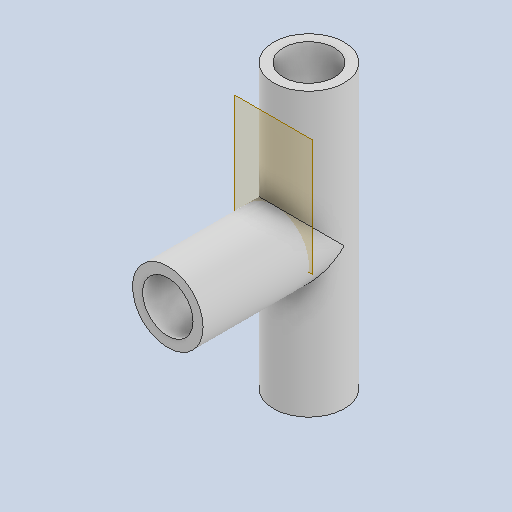
# Autodesk Inventor part: T-joint
Saved by Autodesk Inventor 2025 (Build 290162000, 162)
## iProperties
Created: 2025-07-16
Part Number: T-joint
Material: Generic
Document SubType Name: Modeling
Designer: Pravoslav
Density: 1 g/cm^3
Appearance: Default
Author: Pravoslav
Autodesk Inventor part; units mm, degrees
ref_plane "YZ Plane" through (0, 0, 0) normal (1, 0, 0) x (0, 1, 0)
ref_plane "XZ Plane" through (0, 0, 0) normal (0, 1, 0) x (-1, 0, 0)
sketch "Sketch1" plane through (0, 0, 0) normal (0, 1, 0) x (-1, 0, 0)
  circle A0 centre (0, 0) radius 3.575
  circle A1 centre (0, 0) radius 5
  dimension "d0" = 7.15
  dimension "d1" = 10
  constraints: 2 centre point, 2 coincident
  measures "d0" diameter of A0
  measures "d1" diameter of A1
extrude "Extrusion1" add sketch "Sketch1" along normal mid plane 40
ref_plane "Work Plane1" through (0, 0, 5) normal (0, 0, 1) x (1, 0, 0)
sketch "Sketch2" plane through (0, 0, 5) normal (0, 0, 1) x (1, 0, 0)
  circle A0 centre (0, 0) radius 3.575
  circle A1 centre (0, 0) radius 5
  line L0 (5, 20) -> (-5, 20) projected
  dimension "d4" = 7.15
  dimension "d5" = 10
  dimension "d22" = 0
  constraints: 2 centre point, 1 coincident
  measures "d4" diameter of A0
  measures "d5" diameter of A1
  measures "d22" distance of point (0, 0) A0.centre
extrude "Extrusion2" add sketch "Sketch2" along normal blind 15 and the other way blind 5
sketch "Sketch3" plane through (0, 0, 20) normal (0, 0, 1) x (1, 0, 0)
  circle A0 centre (0, 0) radius 3.575
  constraints: 1 centre point, 1 coincident
extrude "Extrusion3" cut sketch "Sketch3" against normal up to surface
sketch "Sketch4" plane through (0, 20, 0) normal (0, 1, 0) x (1, 0, 0)
  circle A0 centre (0, 0) radius 3.615
  dimension "d13" = 7.23
  constraints: 1 centre point, 1 coincident
  measures "d13" diameter of A0
extrude "Extrusion4" cut sketch "Sketch4" against normal through all
sketch "Sketch5" plane through (0, 0, -5) normal (0, 0, 1) x (1, 0, 0)
  line L0 (5, 15) -> (-5, 15) projected
  line L1 (-5, -15) -> (5, -15) projected
  line L2 (2, 15) -> (-2, 15)
  line L3 (-2, 15) -> (-2, -15)
  line L4 (-2, -15) -> (2, -15)
  line L5 (2, -15) -> (2, 15)
  point P0 (0, 0)
  dimension "d16" = 4
  dimension "d17" = 2
  constraints: 8 end point, 2 parallel, 2 point on line, 1 horizontal, 1 perpendicular
  measures "d16" distance between parallel lines of L3 L5
  measures "d17" distance from line of point (0, 0) L5
body "Solid1"
